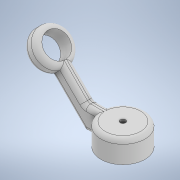
# Autodesk Inventor part: Skrzynia-gora-ramie
Saved by Autodesk Inventor 2022 (Build 260153000, 153)
## iProperties
Created: 2022-03-27
Part Number: Skrzynia-gora-ramie
Material: Ogólny
Document SubType Name: Modeling
Designer: jolow
Density: 1 g/cm^3
Appearance: Domyślna
Author: jolow
Autodesk Inventor part; units mm, degrees
ref_plane "YZ Plane" through (0, 0, 0) normal (1, 0, 0) x (0, 1, 0)
ref_plane "XZ Plane" through (0, 0, 0) normal (0, 1, 0) x (-1, 0, 0)
ref_plane "XY Plane" through (0, 0, 0) normal (0, 0, 1) x (1, 0, 0)
sketch "Szkic1" plane through (0, 0, 0) normal (0, 1, 0) x (-1, 0, 0)
  circle A0 centre (0, 0) radius 20
  dimension "d0" = 40
  constraints: 1 centre point, 1 coincident
  measures "d0" diameter of A0
extrude "Wyciągnięcie proste1" add sketch "Szkic1" along normal mid plane 20
sketch "Szkic2" plane through (0, 0, 0) normal (0, 0, 1) x (1, 0, 0)
  line L0 (-20, -10) -> (20, -10) projected
  line L1 (0, -10) -> (-30, -10)
  line L2 (-30, -10) -> (-30, 10)
  line L3 (-30, 10) -> (0, 10)
  line L4 (0, 10) -> (0, -10)
  line L5 (-30, 10) -> (-60, 40)
  line L6 (-60, 40) -> (-70, 30)
  line L7 (-70, 30) -> (-30, -10)
  line L8 (0, 10) -> (0, 100)
  line L9 (0, 100) -> (-60, 40)
  point P0 (0, 0)
  dimension "d4" = 30
  dimension "d5" = 20
  dimension "d6" = 45
  dimension "d9" = 90
  dimension "d26" = 84.8528
  constraints: 18 end point, 3 parallel, 3 perpendicular, 1 horizontal, 1 midpoint, 1 vertical
  measures "d4" distance of L2.end L3.end
  measures "d5" distance of L1.end L2.end
  measures "d6" angle of L9 L8
  measures "d9" distance of L3.end L8.end
  measures "d26" distance of L8.end L5.end
extrude "Wyciągnięcie proste2" add sketch "Szkic2" along normal mid plane 10 contours L1 L2 L3 L4 L0 | L7 L6 L5 L2
sketch "Szkic3" plane through (-60, 40, 5) normal (0.7071068, 0.7071068, 0) x (0.7071068, -0.7071068, 0)
  line L0 (0, 10) -> (0, 0) projected
  circle A0 centre (0, 5) radius 11
  circle A1 centre (0, 5) radius 16
  point P0 (70.7107, 5)
  dimension "d10" = 22
  dimension "d11" = 5
  constraints: 2 centre point, 1 coincident, 1 midpoint
  measures "d10" diameter of A0
  measures "d11" radial gap between concentric circles of A1 A0
extrude "Wyciągnięcie proste3" add sketch "Szkic3" against normal up to surface (14.1421 mm away)
sketch "Szkic4" plane through (-30, 10, 5) normal (0.7071068, 0.7071068, 0) x (0.7071068, -0.7071068, 0)
  line L0 (-42.4264, 10) -> (-42.4264, 0) projected
  circle A0 centre (-42.4264, 5) radius 11
  point P0 (28.2843, 5)
  constraints: 1 centre point, 1 midpoint
extrude "Wyciągnięcie proste4" cut sketch "Szkic4" against normal through all
sketch "Szkic6" plane through (0, -10, 0) normal (0, -1, 0) x (1, 0, 0)
  circle A0 centre (0, 0) radius 15
  dimension "d19" = 30
  constraints: 1 centre point, 1 coincident
  measures "d19" diameter of A0
extrude "Wyciągnięcie proste6" cut sketch "Szkic6" against normal blind 10
fillet "Zaokrąglenie1" radius 4 12 edges at (20, 10, 0) (-24.6825, 10, 5) (-24.6825, 10, -5) (-30, 10, 0) (-39.6265, 19.6265, -5) (-39.6265, 19.6265, 5) (-81.3137, 41.3137, 0) (-44.6265, 4.6265, 5) (-44.6265, 4.6265, -5) (-30, -10, 0) (-24.6825, -10, 5) (-24.6825, -10, -5)
sketch "Szkic7" plane through (0, 0, 0) normal (0, -1, 0) x (1, 0, 0)
  circle A0 centre (0, 0) radius 7.5
  dimension "d23" = 15
  constraints: 1 centre point, 1 coincident
  measures "d23" diameter of A0
extrude "Wyciągnięcie proste7" cut sketch "Szkic7" against normal blind 5
fillet "Zaokrąglenie2" radius 5 1 edges at (-71.3137, 51.3137, 0)
sketch "Szkic8" plane through (0, 5, 0) normal (0, -1, 0) x (1, 0, 0)
  circle A0 centre (0, 0) radius 2.5
  dimension "d28" = 5
  constraints: 1 centre point, 1 coincident
  measures "d28" diameter of A0
extrude "Wyciągnięcie proste8" cut sketch "Szkic8" against normal blind 10
